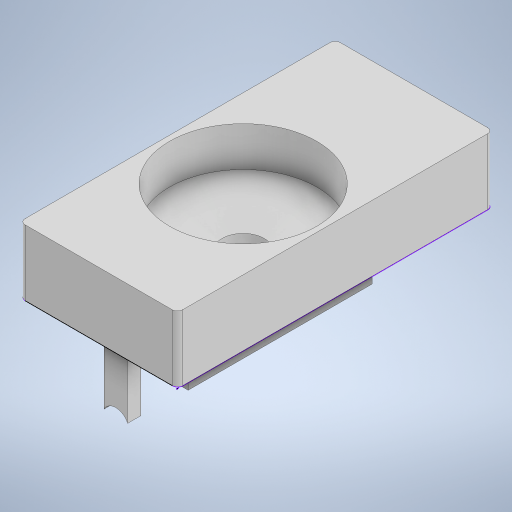
# Autodesk Inventor part: housing_lid_V3
Saved by Autodesk Inventor 2023 (Build 270158000, 158)
## iProperties
Created: 2023-03-23
Part Number: housing_lid_V3
Material: Generic
Document SubType Name: Modeling
Designer: caleb
Density: 1 g/cm^3
Appearance: Default
Author: caleb
## iProperties of the stored document housing_lid_V3_3DPrint.ipt
Created: 2023-04-12
Part Number: housing_lid_V3_3DPrint
Material: Generic
Document SubType Name: Modeling
Designer: czapa
Density: 1 g/cm^3
Appearance: Default
Author: czapa
Autodesk Inventor part; units mm, degrees
sketch "Sketch1" plane through (0, 0, 0) normal (0, 1, 0) x (-1, 0, 0)
  line L0 (0, 0) -> (60, 0)
  line L1 (60, 0) -> (60, -120)
  line L2 (60, -120) -> (0, -120)
  line L3 (0, -120) -> (0, 0)
  line L4 (30, -120) -> (30, 0)
  circle A0 centre (30, -55) radius 22.5
  line L5 (19.5, -90) -> (19.5, -115)
  line L6 (19.5, -115) -> (40.5, -115)
  line L7 (40.5, -115) -> (40.5, -90)
  line L8 (40.5, -90) -> (19.5, -90)
  line L9 (19.5, -90) -> (40.5, -115) construction
  line L10 (19.5, -115) -> (40.5, -90) construction
  line L11 (19.5, -90) -> (44.5, -90) construction
  line L12 (25, -80) -> (25, -90)
  line L13 (25, -90) -> (35, -90)
  line L14 (35, -90) -> (35, -80)
  line L15 (35, -80) -> (25, -80)
  line L16 (25, -80) -> (35, -90) construction
  line L17 (25, -90) -> (35, -80) construction
  line L18 (25, -80) -> (35, -80) construction
  line L19 (7.5, -10) -> (7.5, -80)
  line L20 (7.5, -80) -> (52.5, -80)
  line L21 (52.5, -80) -> (52.5, -10)
  line L22 (52.5, -10) -> (7.5, -10)
  line L23 (7.5, -10) -> (52.5, -80) construction
  line L24 (7.5, -80) -> (52.5, -10) construction
  line L25 (7.5, -10) -> (77.5, -10) construction
  point P0 (30, -115)
  point P1 (30, -90)
  point P2 (30, -90)
  point P3 (30, -80)
  point P4 (30, -77.5)
  point P5 (30, -25)
  point P6 (30, -102.5)
  point P7 (30, -10)
  point P8 (30, -85)
  point P9 (30, -10)
  point P10 (30, -45)
  point P11 (25, -90)
  point P12 (35, -90)
  point P13 (35, -80)
  point P14 (25, -80)
  dimension "d0" = 60
  dimension "d1" = 120
  dimension "d2" = 45
  dimension "d3" = 5
  dimension "d4" = 25
  dimension "d5" = 0
  dimension "d6" = 12.5
  dimension "d7" = 10
  dimension "d8" = 2.5
  dimension "d9" = 22.5
  dimension "d10" = -70
  dimension "d11" = 25
  dimension "d12" = 90
  dimension "d13" = 21
  dimension "d14" = 5
  dimension "d15" = 10
  dimension "d16" = 90
  dimension "d17" = 10
  dimension "d19" = -70
  dimension "d20" = 90
  dimension "d21" = -35
  dimension "d22" = 45
  constraints: 52 end point, 11 parallel, 8 midpoint, 7 perpendicular, 5 point on line, 4 horizontal, 2 coincident, 1 centre point
  measures "d0" distance of L1.end L2.end
  measures "d1" distance of L0.end L1.end
  measures "d2" diameter of A0
  measures "d3" distance from line of L2 point (30, -115)
  measures "d4" distance of point (30, -90) point (30, -115)
  measures "d5" distance of point (30, -90) point (30, -90)
  measures "d6" distance of point (30, -115) point (30, -102.5)
  measures "d7" distance of point (30, -80) point (30, -90)
  measures "d8" distance of point (30, -77.5) point (30, -80)
  measures "d9" distance of point (30, -55) point (30, -77.5)
  measures "d10" distance of point (30, -10) point (30, -80)
  measures "d11" distance of L5.start L5.end
  measures "d12" angle of L5 L11
  measures "d13" distance of L6.end L5.end
  measures "d14" distance of point (30, -85) point (30, -90)
  measures "d15" distance of L12.start L12.end
  measures "d16" angle of L12 L18
  measures "d17" distance of L13.end L12.end
  measures "d19" distance of L19.start L19.end
  measures "d20" angle of L19 L25
  measures "d21" distance of point (30, -80) point (30, -45)
  measures "d22" distance between parallel lines of L19 L21
extrude "Extrusion1" add sketch "Sketch1" along normal blind 20
ref_plane "Work Plane1" through (0, 20, -120) normal (0, 0, -1) x (-1, 0, 0)
sketch "Sketch2" plane through (0, 20, -120) normal (0, 0, -1) x (-1, 0, 0)
  line L0 (0, -20) -> (60, -20) projected
  line L1 (60, -20) -> (60, 0) projected
  line L2 (0, 0) -> (60, 0) projected
  line L3 (0, -20) -> (0, 0) projected
  line L4 (60, -20) -> (0, -20) projected
  line L5 (0, -20) -> (60, -20)
  line L6 (60, -20) -> (60, -80)
  line L7 (60, -80) -> (0, -80)
  line L8 (0, -80) -> (0, -20)
  point P0 (30, -50)
  dimension "d25" = 60
  dimension "d26" = 60
  dimension "d27" = 30
  dimension "d28" = 30
  constraints: 8 end point, 2 parallel, 1 horizontal, 1 perpendicular
  measures "d25" distance of L6.end L7.end
  measures "d26" distance of L5.end L6.end
  measures "d27" distance from line of L7 point (30, -50)
  measures "d28" distance from line of L6 point (30, -50)
ref_plane "Work Plane2" through (-30, -30, -120) normal (0, 1, 0) x (1, 0, 0)
extrude "Extrusion2" add sketch "Sketch1" against normal up to surface (30 mm away) contours L22 L21 A0 L4 | L4 A0 L19 L22 | A0 L4 | L4 A0 | L6 L5 L8 L4 | L4 L8 L7 L6 | A0 L21 L20 L15 L4 | L4 L15 L20 L19 A0 | L8 L12 L15 L4 | L4 L15 L14 L8
extrude "Extrusion3" cut sketch "Sketch1" along normal through all both and the other way through all contours A0 L4 | L4 A0
ref_plane "Work Plane6" through (-7.5, -30, -10) normal (0, 0, -1) x (-1, 0, 0)
ref_plane "Work Plane5" through (-7.5, -30, -80) normal (0, 0, -1) x (-1, 0, 0)
sketch "Sketch3" plane through (-40.5, -30, -115) normal (0, 0, -1) x (-1, 0, 0)
  line L0 (0, 30) -> (0, 0) projected
  circle A0 centre (-10.5, 0) radius 10.5
  point P0 (-40.5, 30)
  constraints: 1 coincident, 1 horizontal alignment, 2 other
sketch "Sketch4" plane through (-19.5, -30, -90) normal (0, 0, -1) x (-1, 0, 0)
  line L0 (5.5, 30) -> (5.5, 0) projected
  line L1 (15.5, 30) -> (15.5, 0) projected
  circle A0 centre (10.5, 0) radius 5
  point P0 (-19.5, 30)
  constraints: 1 coincident, 1 horizontal alignment, 2 other
sketch "Sketch5" plane through (-7.5, -30, -80) normal (0, 0, -1) x (-1, 0, 0)
  line L0 (0, 50) -> (45, 50) projected
  circle A0 centre (22.5, 0) radius 22.5
  point P0 (-7.5, 30)
  constraints: 1 centre point, 1 coincident
extrude "Extrusion4" cut sketch "Sketch3" against normal up to surface (25 mm away)
extrude "Extrusion5" cut sketch "Sketch5" against normal up to surface (70 mm away)
extrude "Extrusion6" cut sketch "Sketch4" against normal up to surface (10 mm away)
sketch "Sketch7" plane through (0, 20, 0) normal (0, 1, 0) x (1, 0, 0)
  circle A0 centre (-30, 55) radius 22.5 projected
  line L0 (-60, 120) -> (-60, 0) projected
  line L1 (-60, 0) -> (0, 0) projected
  line L2 (0, 0) -> (0, 120) projected
  line L3 (0, 120) -> (-60, 120) projected
extrude "Extrusion7" add sketch "Sketch7" along normal blind 5
ref_plane "Work Plane7" through (-30, 0, 0) normal (1, 0, 0) x (0, 0, -1)
sketch "Sketch8" plane through (-30, 0, 0) normal (1, 0, 0) x (0, 0, -1)
  line L0 (0, 0) -> (120, 0) projected
  line L1 (120, 0) -> (120, 25) projected
  line L2 (0, 25) -> (120, 25) projected
  line L3 (0, 0) -> (0, 25) projected
  line L4 (55, -30) -> (55, 0) projected
  line L5 (55, 0) -> (63, 0)
  line L6 (32.5, 25) -> (77.5, 25) projected
  line L7 (55, -30) -> (55, -30) projected
  line L8 (55, -30) -> (55, 0) projected
  line L9 (55, -30) -> (55, -30) projected
  line L10 (55, -30) -> (55, 0) projected
  line L11 (77.5, -7.5) -> (77.5, 25) projected
  line L12 (77.5, 0) -> (77.5, 8)
  line L13 (63, 0) -> (63, 3)
  line L14 (63, 3) -> (77.5, 8)
  dimension "d43" = 8
  dimension "d44" = 8
  dimension "d46" = 3
  constraints: 8 end point, 4 point on line, 1 vertical
  measures "d43" distance of L4.end L5.end
  measures "d44" distance of L12.start L12.end
  measures "d46" distance of L5.end L13.end
revolve "Revolution2" add sketch "Sketch8" angle 360 about axis through (-30, -30, -55) along (0, 1, 0) contours L13 L14 L11 L0
sketch "Sketch9" plane through (0, 25, 0) normal (0, 1, 0) x (1, 0, 0)
  circle A0 centre (-30, 55) radius 22.5 projected
  circle A1 centre (-30, 55) radius 28
  point P0 (0, 0)
  dimension "d48" = 56
  constraints: 1 centre point, 1 coincident
  measures "d48" diameter of A1
extrude "Extrusion8" cut sketch "Sketch9" against normal up to surface round surface about axis through (-30, 5.5, -55) along (0, 1, 0) radius 15.25 half angle 70.974394 far side no
fillet "Fillet1" radius 2 4 edges at (0, 12.5, 0) (0, 12.5, -120) (-60, 12.5, -120) (-60, 12.5, 0)
sketch "Sketch10" plane through (-58, 0, 0) normal (0, 0, 1) x (1, 0, 0)
  line L0 (5.5, -30) -> (5.5, 0) projected
  arc A0 (50.5, -30) -> (5.5, -30) centre (28, -30) ccw projected
  line L1 (5.5, 0) -> (50.5, 0)
  line L2 (50.5, 0) -> (50.5, -30)
  line L3 (50.5, -30) -> (5.5, -30)
  line L4 (5.5, -30) -> (5.5, 0)
  point P0 (58, 0)
  constraints: 8 end point, 2 parallel, 1 horizontal, 1 perpendicular
extrude "Extrusion9" cut sketch "Sketch10" against normal through all
sketch "Sketch11" plane through (0, 0, 0) normal (0, -1, 0) x (1, 0, 0)
  line L0 (-57.9339, 0) -> (-1.9339, 0)
  line L1 (-34.9546, -89.0002) -> (-40.4339, -89.0002)
  line L2 (-40.4339, -89.0002) -> (-40.4339, -90.0002)
  line L3 (-40.4339, -90.0002) -> (-40.5008, -90.0002)
  line L4 (-40.5008, -90.0002) -> (-40.5008, -115.0002)
  line L5 (-40.5008, -115.0002) -> (-40.4339, -115.0002)
  line L6 (-40.4339, -115.0002) -> (-40.4339, -116.0002)
  line L7 (-40.4339, -116.0002) -> (-35.9339, -116.0002)
  line L8 (-35.9339, -116.0002) -> (-35.9339, -120)
  line L9 (-35.9339, -120) -> (-57.9339, -120)
  arc A0 (-59.9339, -118) -> (-57.9339, -120) centre (-57.9339, -118) ccw
  line L10 (-59.9339, -118) -> (-59.9339, -2)
  arc A1 (-57.9339, 0) -> (-59.9339, -2) centre (-57.9339, -2) ccw
  arc A2 (0.0661, -2) -> (-1.9339, 0) centre (-1.9339, -2) ccw
  line L11 (0.0661, -2) -> (0.0661, -118)
  arc A3 (-1.9339, -120) -> (0.0661, -118) centre (-1.9339, -118) ccw
  line L12 (-1.9339, -120) -> (-23.9339, -120)
  line L13 (-23.9339, -120) -> (-23.9339, -116.0002)
  line L14 (-23.9339, -116.0002) -> (-19.5008, -116.0002)
  line L15 (-19.5008, -116.0002) -> (-19.5008, -89.0002)
  line L16 (-19.5008, -89.0002) -> (-24.9546, -89.0002)
  line L17 (-24.9546, -89.0002) -> (-24.9546, -82.005)
  line L18 (-24.9546, -82.005) -> (-6.9339, -82.005)
  line L19 (-6.9339, -82.005) -> (-6.9339, -11.005)
  line L20 (-6.9339, -11.005) -> (-24.9546, -11.005)
  line L21 (-24.9546, -11.005) -> (-24.9546, -6.005)
  line L22 (-24.9546, -6.005) -> (-34.9546, -6.005)
  line L23 (-34.9546, -11.005) -> (-34.9546, -6.005)
  line L24 (-34.9546, -11.005) -> (-52.9339, -11.005)
  line L25 (-52.9339, -11.005) -> (-52.9339, -82.005)
  line L26 (-52.9339, -82.005) -> (-34.9546, -82.005)
  line L27 (-34.9546, -82.005) -> (-34.9546, -89.0002)
  line L28 (-35.9339, -120) -> (-23.9339, -120)
  line L29 (-58, 0) -> (-2, 0) projected
  point P0 (0, 0)
  point P1 (0, 0.3035)
  point P2 (0, 0)
  point P3 (0, -0.3035)
  constraints: 58 end point, 8 point on circle, 4 centre point, 2 symmetric about line, 1 collinear
sketch "Sketch13" plane through (0, 0, 0) normal (0, -1, 0) x (1, 0, 0)
  line L0 (-57.9339, 0) -> (-1.9339, 0)
  line L1 (-40.5008, -115.0002) -> (-40.4339, -115.0002)
  line L2 (-40.4339, -115.0002) -> (-40.4339, -116.0002)
  line L3 (-40.4339, -116.0002) -> (-35.9339, -116.0002)
  line L4 (-35.9339, -116.0002) -> (-35.9339, -120)
  line L5 (-35.9339, -120) -> (-57.9339, -120)
  arc A0 (-59.9339, -118) -> (-57.9339, -120) centre (-57.9339, -118) ccw
  line L6 (-23.9339, -120) -> (-23.9339, -116.0002)
  line L7 (-35.9339, -120) -> (-23.9339, -120)
  line L8 (-52.9339, -82.005) -> (-34.9546, -82.005)
  line L9 (-40.5008, -90.0002) -> (-40.5008, -115.0002)
  line L10 (-19.5008, -116.0002) -> (-19.5008, -89.0002)
  line L11 (-40.4339, -89.0002) -> (-40.4339, -90.0002)
  line L12 (-34.9546, -89.0002) -> (-40.4339, -89.0002)
  line L13 (-34.9546, -82.005) -> (-34.9546, -89.0002)
  line L14 (-19.5008, -89.0002) -> (-24.9546, -89.0002)
  line L15 (-24.9546, -89.0002) -> (-24.9546, -82.005)
  line L16 (-24.9546, -82.005) -> (-6.9339, -82.005)
  line L17 (-40.4339, -90.0002) -> (-40.5008, -90.0002)
  line L18 (-1.9339, -120) -> (-23.9339, -120)
  arc A1 (-1.9339, -120) -> (0.0661, -118) centre (-1.9339, -118) ccw
  line L19 (-59.9339, -118) -> (-59.9339, -2)
  line L20 (0.0661, -2) -> (0.0661, -118)
  line L21 (-6.9339, -82.005) -> (-6.9339, -11.005)
  line L22 (-52.9339, -11.005) -> (-52.9339, -82.005)
  line L23 (-34.9546, -11.005) -> (-52.9339, -11.005)
  line L24 (-34.9546, -11.005) -> (-34.9546, -6.005)
  line L25 (-24.9546, -11.005) -> (-24.9546, -6.005)
  line L26 (-24.9546, -6.005) -> (-34.9546, -6.005)
  arc A2 (-57.9339, 0) -> (-59.9339, -2) centre (-57.9339, -2) ccw
  arc A3 (0.0661, -2) -> (-1.9339, 0) centre (-1.9339, -2) ccw
  line L27 (-6.9339, -11.005) -> (-24.9546, -11.005)
  line L28 (-23.9339, -116.0002) -> (-19.5008, -116.0002)
  line L29 (-58, 0) -> (-2, 0)
  line L30 (-24.9546, -89.0002) -> (-25.4546, -89.0002)
  line L31 (-34.4546, -89.0002) -> (-34.4546, -82.005)
  line L32 (-25.4546, -82.005) -> (-25.4546, -89.0002)
  line L33 (-24.9546, -11.005) -> (-25.4546, -11.005)
  line L34 (-25.4546, -11.005) -> (-25.4546, -10.505)
  line L35 (-34.9546, -6.005) -> (-34.4546, -6.005)
  line L36 (-34.4546, -6.005) -> (-34.4546, -6.505)
  line L37 (-34.4546, -6.505) -> (-34.9546, -6.505)
  line L38 (-34.9546, -6.505) -> (-34.9546, -6.005)
  line L39 (-34.4546, -10.505) -> (-34.4546, -6.505)
  line L40 (-34.4546, -6.505) -> (-25.4546, -6.505)
  line L41 (-25.4546, -6.505) -> (-25.4546, -10.505)
  line L42 (-34.4546, -82.005) -> (-34.4546, -81.505)
  line L43 (-34.4546, -81.505) -> (-25.4546, -81.505)
  line L44 (-25.4546, -81.505) -> (-25.4546, -82.005)
  line L45 (-34.4546, -10.505) -> (-34.4546, -11.005)
  line L46 (-25.4546, -10.505) -> (-25.4546, -11.505)
  line L47 (-25.4546, -11.505) -> (-34.4546, -11.505)
  line L48 (-34.4546, -11.505) -> (-34.4546, -10.505)
  line L49 (-34.4546, -89.0002) -> (-34.4546, -89.5002)
  line L50 (-34.4546, -89.5002) -> (-25.4546, -89.5002)
  line L51 (-25.4546, -89.5002) -> (-25.4546, -89.0002)
  point P0 (0, 0)
  point P1 (0, 0)
  point P2 (0, 0.3035)
  point P3 (0, 0)
  point P4 (0, -0.3035)
  dimension "d54" = 0.5
  dimension "d55" = 0.5
  dimension "d56" = 0.5
  dimension "d57" = 0.5
  dimension "d58" = 0.5
  dimension "d59" = 0.5
  dimension "d73" = 0.5
  dimension "d74" = 1
  dimension "d102" = 0.5
  constraints: 104 end point, 8 point on circle, 5 parallel, 4 centre point, 4 perpendicular, 4 vertical, 3 horizontal, 2 symmetric about line, 1 collinear
  measures "d54" distance of L14.end L30.end
  measures "d55" distance of L8.end L31.end
  measures "d56" distance of L25.start L33.end
  measures "d57" distance of L33.end L34.end
  measures "d58" distance of L36.end L37.end
  measures "d59" distance of L35.end L36.end
  measures "d73" distance of L31.end L42.end
  measures "d74" distance of L46.start L46.end
  measures "d102" distance of L31.start L49.end
ref_plane "Work Plane8" through (-34.4546, 0, -6.505) normal (0, 0, 1) x (1, 0, 0)
sketch "Sketch14" plane through (-34.4546, 0, -6.505) normal (0, 0, 1) x (1, 0, 0)
  circle A0 centre (4.4546, -29.5) radius 5
  line L0 (-0.5454, -29.5) -> (-0.5454, -34.5)
  line L1 (9.4546, -34.5) -> (9.4546, -29.5)
  line L2 (-0.5454, -34.5) -> (9.4546, -34.5)
  line L3 (9.4546, -34.5) -> (9.4546, -39.5)
  line L4 (9.4546, -39.5) -> (-0.5454, -39.5)
  line L5 (-0.5454, -39.5) -> (-0.5454, -34.5)
  dimension "d116" = 10
  dimension "d117" = 5
  constraints: 12 end point, 2 parallel, 2 point on circle, 2 tangent, 1 centre point, 1 horizontal, 1 perpendicular, 1 vertical
  measures "d116" diameter of A0
  measures "d117" distance of L2.end L3.end
extrude "Extrusion12" add sketch "Sketch13" along normal blind 35 contours L46 L47 L48 L45 L39 L40 L41 L34 | L31 L42 L43 L44 L32 L51 L50 L49
sketch "Sketch16" plane through (0, 0, 0) normal (0, -1, 0) x (1, 0, 0)
  line L0 (-6.9339, -82.005) -> (-6.9339, -11.005) projected
  line L1 (-52.9339, -11.005) -> (-52.9339, -82.005) projected
  line L2 (-6.9339, -11.005) -> (-7.4339, -11.005)
  line L3 (-7.4339, -11.005) -> (-7.4339, -11.505)
  line L4 (-7.4339, -11.505) -> (-6.9339, -11.505)
  line L5 (-6.9339, -11.505) -> (-6.9339, -11.005)
  line L6 (-52.9339, -82.005) -> (-52.4339, -82.005)
  line L7 (-52.4339, -82.005) -> (-52.4339, -81.505)
  line L8 (-52.4339, -81.505) -> (-52.9339, -81.505)
  line L9 (-52.9339, -81.505) -> (-52.9339, -82.005)
  line L10 (-7.4339, -11.505) -> (-52.4339, -11.505)
  line L11 (-52.4339, -11.505) -> (-52.4339, -81.505)
  line L12 (-52.4339, -81.505) -> (-7.4339, -81.505)
  line L13 (-7.4339, -81.505) -> (-7.4339, -11.505)
  dimension "d120" = 0.5
  dimension "d121" = 0.5
  dimension "d122" = 0.5
  dimension "d123" = 0.5
  constraints: 24 end point, 6 parallel, 3 horizontal, 3 perpendicular
  measures "d120" distance of L4.end L3.end
  measures "d121" distance of L3.end L2.end
  measures "d122" distance of L8.end L7.end
  measures "d123" distance of L7.end L6.end
extrude "Extrusion14" add sketch "Sketch16" along normal blind 30 contours L13 L12 L11 L10
sketch "Sketch20" plane through (-25.4546, 0, -11.505) normal (0, 0, 1) x (1, 0, 0)
  line L0 (-26.9793, 0) -> (-26.9793, -30) projected
  line L1 (18.0207, 0) -> (18.0207, -30) projected
  line L2 (-26.9793, 0) -> (18.0207, 0)
  line L3 (18.0207, 0) -> (18.0207, -10)
  line L4 (18.0207, -10) -> (-26.9793, -10)
  line L5 (-26.9793, -10) -> (-26.9793, 0)
  line L6 (23.4546, 0) -> (-32.5454, 0) projected
  line L7 (-4.5454, 0) -> (-4.5454, -30)
  circle A0 centre (-4.5454, -30) radius 23
  point P0 (6.8124, -10)
  point P1 (-15.9032, -10)
  point P2 (-26.9793, -24.9285)
  point P3 (18.0207, -25.5535)
  dimension "d124" = 10
  dimension "d125" = 30
  dimension "d126" = 46
  constraints: 10 end point, 2 parallel, 1 centre point, 1 coincident, 1 horizontal, 1 midpoint, 1 perpendicular, 1 point on line, 1 vertical
  measures "d124" distance of L2.end L3.end
  measures "d125" distance of L7.start L7.end
  measures "d126" diameter of A0
extrude "Extrusion15" cut sketch "Sketch20" against normal up to surface (70 mm away) contours L4 A0 L0 | A0 L4 | A0 L7 L4 | A0 L4 L7 | L1 A0 L4
sketch "Sketch22" plane through (0, 0, 0) normal (0, -1, 0) x (1, 0, 0)
  line L0 (-19.5008, -116.0002) -> (-19.5008, -89.0002) projected
  line L1 (-19.5008, -89.0002) -> (-24.9546, -89.0002) projected
  line L2 (-40.4339, -116.0002) -> (-35.9339, -116.0002) projected
  line L3 (-40.5008, -90.0002) -> (-40.5008, -115.0002) projected
  line L4 (-40.5008, -115.0002) -> (-40.5008, -116.0002)
  line L5 (-40.5008, -116.0002) -> (-40.0008, -116.0002)
  line L6 (-40.0008, -116.0002) -> (-40.0008, -115.5002)
  line L7 (-40.0008, -115.5002) -> (-40.5008, -115.5002)
  line L8 (-40.5008, -115.5002) -> (-40.5008, -116.0002)
  line L9 (-19.5008, -89.0002) -> (-20.0008, -89.0002)
  line L10 (-20.0008, -89.0002) -> (-20.0008, -89.5002)
  line L11 (-20.0008, -89.5002) -> (-19.5008, -89.5002)
  line L12 (-19.5008, -89.5002) -> (-19.5008, -89.0002)
  line L13 (-20.0008, -89.5002) -> (-40.0008, -89.5002)
  line L14 (-40.0008, -89.5002) -> (-40.0008, -115.5002)
  line L15 (-40.0008, -115.5002) -> (-20.0008, -115.5002)
  line L16 (-20.0008, -115.5002) -> (-20.0008, -89.5002)
  point P0 (0, 0)
  dimension "d103" = 0.5
  dimension "d104" = 0.5
  dimension "d105" = 0.5
  dimension "d106" = 0.5
  constraints: 26 end point, 6 parallel, 3 horizontal, 3 perpendicular, 1 vertical
  measures "d103" distance of L7.end L6.end
  measures "d104" distance of L6.end L5.end
  measures "d105" distance of L11.end L10.end
  measures "d106" distance of L10.end L9.end
extrude "Extrusion16" add sketch "Sketch22" along normal blind 30 contours L16 L15 L14 L13
sketch "Sketch23" plane through (-20.0008, 0, -115.5002) normal (0, 0, -1) x (-1, 0, 0)
  arc A0 (5.4537, -7.9445) -> (-0.4746, -10) centre (9.9537, -30.5) ccw projected
  arc A1 (14.4537, -7.9445) -> (5.4537, -7.9445) centre (9.9537, -30.5) ccw projected
  arc A2 (20.3821, -10) -> (14.4537, -7.9445) centre (9.9537, -30.5) ccw projected
  line L0 (20.3821, -10) -> (32.433, -10) projected
  line L1 (32.433, 0) -> (32.433, -10) projected
  line L2 (-12.567, 0) -> (-12.567, -10) projected
  line L3 (-12.567, -10) -> (-0.4746, -10) projected
  line L4 (0, 0) -> (20, 0) projected
  line L5 (0, 0) -> (0, -30) projected
  line L6 (20, -30) -> (0, -30) projected
  line L7 (20, 0) -> (20, -30) projected
  point P0 (-20.0008, 0)
  point P1 (0, -9.7654)
  point P2 (20, -9.8101)
extrude "Extrusion17" cut sketch "Sketch23" against normal up to surface (26 mm away) contours A1 A2 L7 L6 L5 A0
sketch "Sketch24" plane through (-30, 0, -55) normal (0, 1, 0) x (1, 0, 0)
  circle A0 centre (0, 0) radius 8
  point P0 (30, -55)
  constraints: 1 centre point
extrude "Extrusion18" cut sketch "Sketch24" against normal through all
extrude "Extrusion19" cut sketch "Sketch14" against normal through all
ref_plane "Work Plane3" through (-40.5, -30, -115) normal (0, 0, -1) x (-1, 0, 0)
ref_plane "Work Plane4" through (-19.5, -30, -90) normal (0, 0, -1) x (-1, 0, 0)
equation "\"d4\" = d11"
equation "\"d6\" = 0.5 * d4"
equation "\"d7\" = d15"
equation "\"d9\" = 0.5 * d2"
equation "\"d14\" = 0.5 * d7"
equation "\"d19\" = d10"
equation "\"d22\" = d2"
equation "\"d25\" = d0"
equation "\"d26\" = d25"
equation "\"d21\" = 0.5 * d10"
equation "\"d27\" = 0.5 * d26"
equation "\"d28\" = 0.5 * d25"
body "Solid1"
